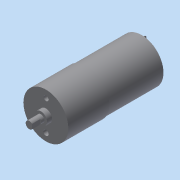
# Autodesk Inventor part: motor
Saved by Autodesk Inventor 2015 (Build 190159000, 159)
## iProperties
Created: 2015-06-23
Part Number: motor
Material: Generic
Document SubType Name: Modeling
Designer: Rahul
Density: 1 g/cm^3
Appearance: Default
Autodesk Inventor part; units mm, degrees
ref_plane "YZ Plane" through (0, 0, 0) normal (1, 0, 0) x (0, 1, 0)
ref_plane "XZ Plane" through (0, 0, 0) normal (0, 1, 0) x (-1, 0, 0)
ref_plane "XY Plane" through (0, 0, 0) normal (0, 0, 1) x (1, 0, 0)
sketch "Sketch1" plane through (0, 0, 0) normal (0, 0, 1) x (1, 0, 0)
  circle A0 centre (0, 0) radius 12.46
  dimension "d0" = 24.92
  constraints: 1 centre point, 1 coincident
  measures "d0" diameter of A0
extrude "Extrusion1" add sketch "Sketch1" along normal blind 22.76
sketch "Sketch2" plane through (0, 0, 22.76) normal (0, 0, 1) x (1, 0, 0)
  circle A0 centre (0, 0) radius 3.43
  arc A1 (1.5, 1.3229) -> (1.5, -1.3229) centre (0, 0) ccw
  line L0 (1.5, -1.3229) -> (1.5, 1.3229)
  dimension "d3" = 6.86
  constraints: 2 centre point, 2 end point, 2 point on circle, 1 coincident, 1 vertical
  measures "d3" diameter of A0
extrude "Extrusion2" add sketch "Sketch2" along normal blind 2.78
extrude "Extrusion3" add sketch "Sketch2" along normal blind 9.22 contours L0 A1
sketch "Sketch3" plane through (0, 0, 25.54) normal (0, 0, 1) x (1, 0, 0)
  circle A0 centre (0, 0) radius 2
  dimension "d12" = 4
  constraints: 1 centre point, 1 coincident
  measures "d12" diameter of A0
extrude "Extrusion4" add sketch "Sketch3" along normal blind 1.85
sketch "Sketch4" plane through (0, 0, 22.76) normal (0, 0, 1) x (1, 0, 0)
  circle A0 centre (0.108, 8.3843) radius 1.385
  circle A1 centre (0, 0) radius 12.46 projected
  circle A2 centre (0, -8.28) radius 1.49
  dimension "d13" = 2.69
  dimension "d14" = 2.77
  dimension "d15" = 2.69
  dimension "d16" = 2.98
  constraints: 2 centre point
  measures "d14" diameter of A0
  measures "d16" diameter of A2
extrude "Extrusion5" cut sketch "Sketch4" against normal blind 5 contours A0
extrude "Extrusion6" cut sketch "Sketch4" against normal blind 5 contours A2
sketch "Sketch10" plane through (0, 0, 0) normal (0, 0, -1) x (-1, 0, 0)
  circle A0 centre (0, 0) radius 12.11
  dimension "d52" = 24.22
  constraints: 1 centre point, 1 coincident
  measures "d52" diameter of A0
sketch "Sketch11" plane through (0, 0, 0) normal (0, 0, -1) x (-1, 0, 0)
  circle A0 centre (0, 0) radius 12.11
  dimension "d53" = 24.22
  constraints: 1 centre point, 1 coincident
  measures "d53" diameter of A0
extrude "Extrusion15" add sketch "Sketch11" along normal blind 30.44
sketch "Sketch14" plane through (0, 0, -30.44) normal (0, 0, -1) x (-1, 0, 0)
  circle A0 centre (0, 0) radius 12.105
  dimension "d59" = 24.21
  constraints: 1 centre point, 1 coincident
  measures "d59" diameter of A0
extrude "Extrusion17" cut sketch "Sketch14" against normal blind 1.05
sketch "Sketch15" plane through (0, 0, -29.39) normal (0, 0, -1) x (-1, 0, 0)
  circle A0 centre (0, 0) radius 3.24
  dimension "d62" = 6.48
  constraints: 1 centre point, 1 coincident
  measures "d62" diameter of A0
extrude "Extrusion18" add sketch "Sketch15" along normal blind 2.31
sketch "Sketch16" plane through (0, 0, -31.7) normal (0, 0, -1) x (-1, 0, 0)
  circle A0 centre (0, 0) radius 3.43 projected
  circle A1 centre (0, 0) radius 1
  dimension "d65" = 2
  constraints: 1 centre point, 1 coincident
  measures "d65" diameter of A1
extrude "Extrusion19" add sketch "Sketch16" along normal blind 3.75 contours A1
fillet "Fillet4" radius 0.5 1 edges at (3.24, 0, -31.7)
sketch "Sketch17" plane through (0, 0, -29.39) normal (0, 0, -1) x (-1, 0, 0)
  line L0 (-0.11, 8.8) -> (0.11, 8.8)
  line L1 (0.11, 8.8) -> (0.11, 10.8)
  line L2 (0.11, 10.8) -> (-0.11, 10.8)
  line L3 (-0.11, 10.8) -> (-0.11, 8.8)
  line L4 (17.444, 0) -> (-17.444, 0) projected
  line L5 (0, -17.444) -> (0, 17.444) projected
  circle A0 centre (0, 0) radius 3.24 projected
  line L6 (-0.11, -10.8) -> (0.11, -10.8)
  line L7 (0.11, -10.8) -> (0.11, -8.8)
  line L8 (0.11, -8.8) -> (-0.11, -8.8)
  line L9 (-0.11, -8.8) -> (-0.11, -10.8)
  dimension "d69" = 2
  dimension "d70" = 0.22
  dimension "d71" = 8.8
  dimension "d72" = 0.22
  dimension "d73" = 2
  dimension "d74" = 8.8
  constraints: 16 end point, 4 parallel, 2 horizontal, 2 perpendicular, 2 other
  measures "d69" distance of L2.end L0.start
  measures "d70" distance of L1.end L2.end
  measures "d71" distance from line of L0 A0.centre
  measures "d72" distance of L7.end L8.end
  measures "d73" distance of L8.end L6.start
  measures "d74" distance from line of L8 point (0, 0)
sketch "Sketch18" plane through (0, 0, -29.39) normal (0, 0, -1) x (-1, 0, 0)
  point P0 (0, 0)
sketch "Sketch19" plane through (0, 0, -29.39) normal (0, 0, -1) x (-1, 0, 0)
  point P0 (0, 0)
extrude "Extrusion20" add sketch "Sketch17" along normal blind 3.54 contours L6 L9 L8 L5 | L5 L8 L7 L6
extrude "Extrusion21" add sketch "Sketch17" along normal blind 3.54 contours L3 L2 L5 L0 | L5 L2 L1 L0
chamfer "Chamfer1" distance 0.6 angle 45 2 edges at (0, -10.8, -32.93) (0, -8.8, -32.93)
chamfer "Chamfer2" distance 0.6 angle 45 2 edges at (0, 10.8, -32.93) (0, 8.8, -32.93)
body "Solid1"
